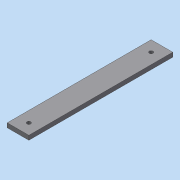
# Autodesk Inventor part: Part3
Saved by Autodesk Inventor 2016 SP1 (Build 200210100, 210)
## iProperties
Created: 2016-03-17
Part Number: Part3
Material: Generic
Document SubType Name: Modeling
Designer: Mohamed A.
Density: 1 g/cm^3
Appearance: Default
Author: Mohamed A.
Autodesk Inventor part; units mm, degrees
ref_plane "YZ Plane" through (0, 0, 0) normal (1, 0, 0) x (0, 1, 0)
ref_plane "XZ Plane" through (0, 0, 0) normal (0, 1, 0) x (-1, 0, 0)
ref_plane "XY Plane" through (0, 0, 0) normal (0, 0, 1) x (1, 0, 0)
sketch "Sketch1" plane through (0, 0, 0) normal (0, 0, 1) x (1, 0, 0)
  line L0 (-7.5, 50) -> (7.5, 50)
  line L1 (7.5, 50) -> (7.5, -50)
  line L2 (7.5, -50) -> (-7.5, -50)
  line L3 (-7.5, -50) -> (-7.5, 50)
  line L4 (-7.5, 50) -> (7.5, -50) construction
  line L5 (7.5, 50) -> (-7.5, -50) construction
  circle A0 centre (0, 42.5) radius 1.35
  circle A1 centre (0, -42.5) radius 1.35
  point P0 (0, 0)
  dimension "d0" = 15
  dimension "d1" = 100
  dimension "d4" = 2.7
  dimension "d5" = 7.5
  dimension "d6" = 2.7
  dimension "d7" = 7.5
  constraints: 12 end point, 2 centre point, 2 midpoint, 2 parallel, 1 horizontal, 1 perpendicular
  measures "d0" distance of L1.end L2.end
  measures "d1" distance of L0.end L1.end
  measures "d4" diameter of A0
  measures "d5" distance from line of A0.centre L0
  measures "d6" diameter of A1
  measures "d7" distance from line of L2 A1.centre
extrude "Extrusion1" add sketch "Sketch1" along normal blind 3
equation "\"d5\" = 0.5 * d0"
equation "\"d7\" = d5"
body "Solid1"
